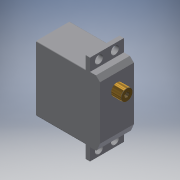
# Autodesk Inventor part: Corona-MG339MG
Saved by Autodesk Inventor 2017 (Build 210142000, 142)
## iProperties
Created: 2014-12-16
Part Number: Corona-MG339MG
Material: Generic
Document SubType Name: Modeling
Designer: Vinicius
Density: 1 g/cm^3
Appearance: Default
Mass: 18.147 g
Surface Area: 48.3885 cm^2
Volume: 18.147 cm^3
Author: Vinicius
Autodesk Inventor part; units mm, degrees
ref_plane "YZ Plane" through (0, 0, 0) normal (1, 0, 0) x (0, 1, 0)
ref_plane "XZ Plane" through (0, 0, 0) normal (0, 1, 0) x (-1, 0, 0)
ref_plane "XY Plane" through (0, 0, 0) normal (0, 0, 1) x (1, 0, 0)
sketch "Sketch1" plane through (0, 0, 0) normal (0, 1, 0) x (-1, 0, 0)
  line L0 (-16, 16.35) -> (16, 16.35)
  line L1 (16, 16.35) -> (16, -16.35)
  line L2 (16, -16.35) -> (-16, -16.35)
  line L3 (-16, -16.35) -> (-16, 16.35)
  line L4 (-16, 16.35) -> (16, -16.35) construction
  line L5 (16, 16.35) -> (-16, -16.35) construction
  point P0 (0, 0)
  dimension "d0" = 32
  dimension "d1" = 32.7
  constraints: 12 end point, 2 midpoint, 2 parallel, 1 horizontal, 1 perpendicular
  measures "d0" distance of L1.end L2.end
  measures "d1" distance of L0.end L1.end
extrude "Extrusion1" add sketch "Sketch1" along normal blind 17
chamfer "Chamfer1" distance 2 angle 45 2 edges at (16, 8.5, 16.35) (16, 8.5, -16.35)
chamfer "Chamfer2" distance 2 angle 45 1 edges at (16, 8.5, -14.35)
sketch "Sketch3" plane through (16, 0, 14.35) normal (1, 0, 0) x (0, 0, -1)
  line L0 (-2, 17) -> (-2, 0) projected
  circle A0 centre (7.2, 8.5) radius 2.9
  point P0 (14.35, 0)
  point P1 (-2, 8.5)
  dimension "d10" = 9.2
  dimension "d11" = 5.8
  constraints: 1 centre point, 1 horizontal alignment, 1 midpoint
  measures "d10" distance from line of L0 A0.centre
  measures "d11" diameter of A0
extrude "Extrusion2" add sketch "Sketch3" along normal blind 5
sketch "Sketch4" plane through (-16, 0, 16.35) normal (0, 0, 1) x (1, 0, 0)
  line L0 (30, 17) -> (0, 17) projected
  line L1 (24.8, 17) -> (27, 17)
  line L2 (27, 17) -> (27, 0)
  line L3 (27, 0) -> (24.8, 0)
  line L4 (24.8, 0) -> (24.8, 17)
  line L5 (32, 0) -> (32, 17) projected
  point P0 (16, 0)
  point P1 (25.9, 0)
  dimension "d14" = 5
  dimension "d15" = 2.2
  constraints: 8 end point, 2 parallel, 1 horizontal, 1 horizontal alignment, 1 midpoint, 1 perpendicular, 1 point on line
  measures "d14" distance between parallel lines of L5 L2
  measures "d15" distance between parallel lines of L4 L2
extrude "Extrusion3" add sketch "Sketch4" along normal blind 6.2
sketch "Sketch5" plane through (11, 0, 16.35) normal (1, 0, 0) x (0, 0, -1)
  line L0 (0, 17) -> (0, 0) projected
  line L1 (0, 17) -> (-6.2, 17) projected
  line L2 (-6.2, 0) -> (-6.2, 17) projected
  line L3 (0, 0) -> (-6.2, 0) projected
  line L4 (0, 17) -> (-6.2, 17) construction
  line L5 (-3.2, 17) -> (-3.2, 12.4994) construction
  line L6 (-3.2, 12.4994) -> (-3.2, 4.4994) construction
  line L7 (-3.2, 4.4994) -> (-3.1, 0) construction
  point P0 (16.35, 0)
  dimension "d18" = 3
  dimension "d19" = 8
  constraints: 6 end point, 1 equal length, 1 midpoint, 1 perpendicular, 1 point on line, 1 vertical, 1 vertical alignment
  measures "d18" distance from line of L2 L6.end
  measures "d19" distance of L6.end L5.end
hole "Hole1" at (11, 12.4994, 19.55) at (11, 4.4994, 19.55) direction (-1, 0, 0) diameter 4 depth 8 tip angle 118
sketch "Sketch6" plane through (-16, 0, -16.35) normal (0, 0, -1) x (-1, 0, 0)
  line L0 (-27, 17) -> (-24.8, 17) projected
  line L1 (-24.8, 17) -> (-24.8, 0) projected
  line L2 (-24.8, 0) -> (-27, 0) projected
  line L3 (-27, 0) -> (-27, 17) projected
  line L4 (-27, 17) -> (-24.8, 17)
  line L5 (-24.8, 17) -> (-24.8, 0)
  line L6 (-24.8, 0) -> (-27, 0)
  line L7 (-27, 0) -> (-27, 17)
  point P0 (-16, 0)
  constraints: 8 end point, 2 parallel, 1 horizontal, 1 perpendicular
extrude "Extrusion4" add sketch "Sketch6" along normal blind 6.2
sketch "Sketch7" plane through (11, 0, -16.35) normal (1, 0, 0) x (0, 0, -1)
  circle A0 centre (-35.9, 12.4994) radius 2 projected
  circle A1 centre (-35.9, 4.4994) radius 2 projected
  line L0 (6.2, 17) -> (6.2, 0) projected
  point P0 (-16.35, 0)
  point P1 (3.2, 12.4994)
  point P2 (3.2, 4.4994)
  dimension "d29" = 3
  constraints: 2 horizontal alignment, 1 vertical alignment
  measures "d29" distance from line of L0 point (3.2, 12.499)
hole "Hole2" at (11, 12.4994, -19.55) at (11, 4.4994, -19.55) direction (-1, 0, 0) diameter 4 depth 8 tip angle 118
chamfer "Chamfer3" distance 0.1 angle 45 1 edges at (21, 8.5, 10.05)
fillet "Fillet1" radius 0.5 4 edges at (-3.6, 17, 16.35) (-3.6, 17, -16.35) (-3.6, 0, 16.35) (-3.6, 0, -16.35)
hole "Hole3" at (21, 8.5, 7.15) direction (-1, 0, 0) diameter 2.459 depth 6 tip angle 118 thread size "M3x0.5" class "6H" standard "ISO Metric profile"
body "Solid1"
